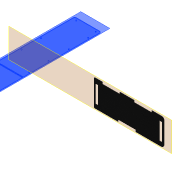
# Autodesk Inventor part: Spacing Layer 3
Saved by Autodesk Inventor 2017 (Build 210142000, 142)
## iProperties
Created: 2016-11-08
Part Number: Spacing Layer 3
Material: PC/ABS Plastic
Document SubType Name: Modeling
Designer: Jonis
Density: 0.357273 g/cm^3
Appearance: Fine Textured - Black
Author: Jonis
Autodesk Inventor part; units mm, degrees
ref_plane "YZ Plane" through (0, 0, 0) normal (1, 0, 0) x (0, 1, 0)
ref_plane "XZ Plane" through (0, 0, 0) normal (0, 1, 0) x (-1, 0, 0)
ref_plane "XY Plane" through (0, 0, 0) normal (0, 0, 1) x (1, 0, 0)
ref_plane "Work Plane1" through (280, 50, 0) normal (0, 0, 1) x (1, 0, 0)
sketch "Sketch3" plane through (280, 50, 0) normal (0, 0, 1) x (1, 0, 0)
  line L0 (280, 39.9924) -> (280, 21.7788) projected
  line L1 (280, 21.7788) -> (280, -15.0258) projected
  line L2 (280, -15.0258) -> (280, -34.9902) projected
  line L3 (280, -34.9902) -> (280, -39.994) projected
  arc A0 (269.9924, -50.0016) -> (280, -39.994) centre (269.9924, -39.994) ccw projected
  arc A1 (280, 39.9924) -> (269.9924, 50) centre (269.9924, 39.9924) ccw projected
  line L4 (242.662, 50) -> (269.9924, 50) projected
  line L5 (269.9924, -50.0016) -> (261.331, -50.0016) projected
  line L6 (261.331, -50.0016) -> (182.2354, -50.0016) projected
  line L7 (98.3122, -50) -> (22.952, -50) projected
  arc A2 (16.0432, -47.46) -> (18.5832, -50) centre (18.5832, -47.46) ccw projected
  line L8 (22.952, -50) -> (18.5832, -50) projected
  line L9 (16.0432, -47.46) -> (16.0432, 32.1674) projected
  line L10 (16.0432, 32.1674) -> (16.0432, 47.46) projected
  arc A3 (18.5832, 50) -> (16.0432, 47.46) centre (18.5832, 47.46) ccw projected
  line L11 (18.5832, 50) -> (37.762, 50) projected
  line L12 (121.9848, 50) -> (155.413, 50) projected
  line L13 (121.9848, 50) -> (37.762, 50)
  line L14 (155.413, 50) -> (242.662, 50)
  line L15 (182.2354, -50.0016) -> (97.9077, -50)
  point P0 (-280, -50)
  constraints: 6 end point, 2 collinear, 1 point on line
extrude "Extrusion2" add sketch "Sketch3" along normal blind 1.6
sketch "Sketch5" plane through (280, 50, 1.6) normal (0, 0, 1) x (1, 0, 0)
  circle A0 centre (263.7186, 35.6472) radius 1.75 projected
  circle A1 centre (250.0026, 44.1308) radius 1.75 projected
  circle A2 centre (263.7186, -38.0128) radius 1.75 projected
  circle A3 centre (250.0026, -44.1088) radius 1.75 projected
  circle A4 centre (176.9522, -44.1088) radius 1.75 projected
  circle A5 centre (163.033, 44.1308) radius 1.75 projected
  circle A6 centre (116.7034, 44.1054) radius 1.75 projected
  circle A7 centre (103.2922, -44.1088) radius 1.75 projected
  circle A8 centre (43.0434, -44.1342) radius 1.75 projected
  circle A9 centre (43.0434, 44.1054) radius 1.75 projected
  circle A10 centre (21.682, 35.6472) radius 1.75 projected
  circle A11 centre (21.682, -38.0128) radius 1.75 projected
  circle A12 centre (236.693, 44.1308) radius 1.75 projected
  point P0 (-280, -50)
hole "Hole1" at (530.0026, 94.1308, 1.6) at (516.693, 94.1308, 1.6) at (543.7186, 85.6472, 1.6) at (543.7186, 11.9872, 1.6) at (530.0026, 5.8912, 1.6) at (443.033, 94.1308, 1.6) at (456.9522, 5.8912, 1.6) at (383.2922, 5.8912, 1.6) at (396.7034, 94.1054, 1.6) at (323.0434, 94.1054, 1.6) at (301.682, 85.6472, 1.6) at (323.0434, 5.8658, 1.6) at (301.682, 11.9872, 1.6) direction (0, 0, -1) diameter 1.6 depth 8 tip angle 118
sketch "Sketch6" plane through (280, 50, 1.6) normal (0, 0, 1) x (1, 0, 0)
  line L0 (262.604, 31.9897) -> (272.504, 31.9897) projected
  line L1 (262.604, 31.9897) -> (262.604, -34.5603) projected
  line L2 (272.504, -34.5603) -> (262.604, -34.5603) projected
  line L3 (173.2947, -42.9941) -> (173.2947, -52.8941) projected
  line L4 (173.2947, -42.9941) -> (106.7447, -42.9941) projected
  line L5 (106.7447, -52.8941) -> (106.7447, -42.9941) projected
  line L6 (30.4674, -34.5603) -> (20.5674, -34.5603) projected
  line L7 (30.4674, 31.9897) -> (30.4674, -34.5603) projected
  line L8 (20.5674, 31.9897) -> (30.4674, 31.9897) projected
  line L9 (46.7009, 42.9907) -> (46.7009, 52.8907) projected
  line L10 (46.7009, 42.9907) -> (113.2509, 42.9907) projected
  line L11 (113.2509, 52.8907) -> (113.2509, 42.9907) projected
  line L12 (166.6906, 43.0161) -> (166.6906, 52.9161) projected
  line L13 (166.6906, 43.0161) -> (233.2406, 43.0161) projected
  line L14 (233.2406, 52.9161) -> (233.2406, 43.0161) projected
  line L15 (166.6906, 52.9161) -> (233.2406, 52.9161) projected
  line L16 (46.7009, 52.8907) -> (113.2509, 52.8907) projected
  line L17 (20.5674, 31.9897) -> (20.5674, -34.5603) projected
  line L18 (173.2947, -52.8941) -> (106.7447, -52.8941) projected
  line L19 (272.504, 31.9897) -> (272.504, -34.5603) projected
  point P0 (-280, -50)
extrude "Extrusion3" cut sketch "Sketch6" against normal blind 1.6
body "Solid2"
